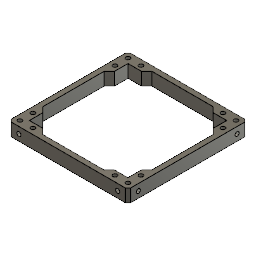
STRUCTURE UPPER FOSSASAT-1 v2 (Autodesk Fusion 360 design; units mm, degrees)
Autodesk Fusion 360 part; units mm, degrees
sketch "Sketch1" plane through (0, 0, 0) normal (0, 1, 0) x (1, 0, 0)
  line L0 (0, 0) -> (46, 0)
  line L1 (46, 0) -> (46, -46)
  line L2 (46, -46) -> (0, -46)
  line L3 (0, -46) -> (0, 0)
  line L4 (0, 0) -> (2, 0)
  line L5 (2, 0) -> (2, -2)
  circle A0 centre (2, -2) radius 0.8
  line L6 (5, -1.5) -> (5, -1)
  line L7 (23, 0) -> (23, -46)
  line L8 (23, -23) -> (42, -23)
  line L9 (42, -23) -> (42, -4)
  line L10 (42, -4) -> (4, -4)
  line L11 (4, -4) -> (4, -42)
  line L12 (4, -42) -> (42, -42)
  line L13 (42, -42) -> (42, -4)
  line L14 (0, -46) -> (2, -46)
  line L15 (2, -46) -> (2, -44)
  circle A1 centre (2, -44) radius 0.8
  line L16 (46, -46) -> (44, -46)
  line L17 (44, -46) -> (44, -44)
  circle A2 centre (44, -44) radius 0.8
  line L18 (46, 0) -> (44, 0)
  line L19 (44, 0) -> (44, -2)
  circle A3 centre (44, -2) radius 0.8
  line L20 (42, -4) -> (45.9628, -7.9628)
  line L21 (42, -4) -> (47.6042, -4) construction
  line L22 (42, -4) -> (38, 0)
  line L23 (42, -42) -> (46, -38)
  line L24 (46, -38) -> (38, -46)
  line L25 (4, -42) -> (8, -46)
  line L26 (8, -46) -> (0, -38)
  line L27 (4, -4) -> (8, 0)
  line L28 (8, 0) -> (0, -8)
  line L29 (2, -39) -> (2, -41)
  line L30 (2, -41) -> (2, -4)
  line L31 (5.0409, -2) -> (42, -2)
  line L32 (4, -44) -> (42, -44)
  line L33 (44, -40.936) -> (44, -4)
  dimension "d1" = 46
  dimension "d2" = 2
  dimension "d3" = 19
  dimension "d4" = 19
  dimension "d5" = 38
  dimension "d6" = 38
  dimension "d7" = 1.6
  dimension "d8" = 2
  dimension "d9" = 45
  measures "d4" distance of L0.start
  measures "d6" distance of L0.start
  measures "d7" diameter of A2
  measures "d9" angle of L20 L21
extrude "Extrude1" add sketch "Sketch1" along normal blind 6 contours L0 L3 L4 L27 L28 | L3 L26 L28 L29 L30 | L0 L7 L27 L28 L31 | L2 L3 L14 L25 L26 | L0 L7 L22 L31 | L0 L1 L18 L20 L22 L23 L24 L33 | L2 L7 L25 L26 L32 | L2 L7 L24 L32 | L1 L2 L16 L23 L24
extrude "Extrude2" cut 1 faces at (45.3333, 6, 14.6667) along direction (0, -1, 0) blind 1
chamfer "Chamfer1" distance 1 angle 45 4 edges at (46, 2.5, 46) (0, 2.5, 46) (46, 2.5, 0) (0, 2.5, 0)
sketch "Sketch2" plane through (0, 0, 0) normal (0, 0, -1) x (-1, 0, 0)
  line L0 (-1, 0) -> (-1, 5)
  line L1 (-1, 5) -> (-45, 5)
  line L2 (-45, 5) -> (-45, 0)
  line L3 (-45, 0) -> (-1, 0)
  line L4 (0, 0) -> (0, 5)
  line L5 (0, 2.5) -> (-4, 2.5)
  circle A0 centre (-4, 2.5) radius 0.8
  line L6 (-46, 5) -> (-46, 0)
  line L7 (-46, 2.5) -> (-42, 2.5)
  circle A1 centre (-42, 2.5) radius 0.8
  dimension "d15" = 1.6
  dimension "d16" = 4
  dimension "d17" = 1.6
  measures "d15" diameter of A0
  measures "d17" diameter of A1
extrude "Extrude3" cut sketch "Sketch2" against normal blind 3 contours A0 | A1
sketch "Sketch3" plane through (0, 0, 0) normal (-1, 0, 0) x (0, 0, 1)
  line L0 (1, 5) -> (1, 0)
  line L1 (1, 0) -> (45, 0)
  line L2 (45, 0) -> (45, 5)
  line L3 (45, 5) -> (1, 5)
  line L4 (0, 2.5) -> (4, 2.5)
  line L5 (46, 5) -> (46, 0)
  line L6 (46, 2.5) -> (42, 2.5)
  circle A0 centre (42, 2.5) radius 0.8
  circle A1 centre (4, 2.5) radius 0.8
  dimension "d20" = 4
  dimension "d21" = 1.6
  dimension "d22" = 1.6
  measures "d21" diameter of A0
  measures "d22" diameter of A1
extrude "Extrude4" cut sketch "Sketch3" against normal blind 3 contours A0 | A1
sketch "Sketch4" plane through (0, 0, 46) normal (0, 0, 1) x (1, 0, 0)
  line L0 (1, 5) -> (1, 0)
  line L1 (1, 0) -> (45, 0)
  line L2 (45, 0) -> (45, 5)
  line L3 (45, 5) -> (1, 5)
  line L4 (0, 2.5) -> (4, 2.5)
  circle A0 centre (4, 2.5) radius 0.8
  line L5 (46, 0) -> (46, 5)
  line L6 (42, 0) -> (42, 5)
  line L7 (46, 2.5) -> (42, 2.5)
  circle A1 centre (42, 2.5) radius 0.8
  dimension "d25" = 1.6
  dimension "d26" = 1.6
  measures "d25" diameter of A0
  measures "d26" diameter of A1
extrude "Extrude5" cut sketch "Sketch4" against normal blind 1.6 contours L6 L7 A1 | L6 A1 | L6 L7 A1 | A0
sketch "Sketch5" plane through (46, 0, 0) normal (1, 0, 0) x (0, 0, -1)
  line L0 (-1, 0) -> (-1, 5)
  line L1 (-1, 5) -> (-45, 5)
  line L2 (-45, 5) -> (-45, 0)
  line L3 (-45, 0) -> (-1, 0)
  line L4 (-46, 2.5) -> (-42, 2.5)
  circle A0 centre (-42, 2.5) radius 0.8
  line L5 (0, 2.5) -> (-4, 2.5)
  circle A1 centre (-4, 2.5) radius 0.8
  dimension "d29" = 4
  dimension "d30" = 1.6
  measures "d30" diameter of A1
extrude "Extrude6" cut sketch "Sketch5" against normal blind 3 contours A0 | A1
extrude "Extrude7" cut 2 faces at (4.3142, 2.6814, 44.4) (42.1333, 2.9623, 44.4) along direction (0, 0, -1) blind 1.4
sketch "Sketch6" plane through (0, 5, 0) normal (0, 1, 0) x (-1, 0, 0)
  circle A0 centre (-2, 2) radius 0.8
  circle A1 centre (-2, 44) radius 0.8
  circle A2 centre (-44, 2) radius 0.8
  circle A3 centre (-44, 44) radius 0.8
  line L0 (-40, 2) -> (-42, 4)
  line L1 (-42, 4) -> (-44, 6)
  line L2 (-44, 6) -> (-44, 40)
  line L3 (-44, 40) -> (-40, 44)
  line L4 (-40, 44) -> (-6, 44)
  line L5 (-6, 44) -> (-2, 40)
  line L6 (-2, 40) -> (-2, 6)
  line L7 (-2, 6) -> (-6, 2)
  line L8 (-6, 2) -> (-40, 2)
  line L9 (-1, 0) -> (0, 1)
  line L10 (0, 1) -> (0, 45)
  line L11 (0, 45) -> (-1, 46)
  line L12 (-1, 46) -> (-45, 46)
  line L13 (-45, 46) -> (-46, 45)
  line L14 (-46, 45) -> (-46, 1)
  line L15 (-46, 1) -> (-45, 0)
  line L16 (-45, 0) -> (-1, 0)
  line L17 (-46, 38.6089) -> (-43.8, 38.6089)
  line L18 (-44, 44) -> (-42, 44)
  line L19 (-43.8, 38.6089) -> (-43.8, 44)
  line L20 (-43.8, 44) -> (-43.8, 39)
  line L21 (-23, 23) -> (-23, 42)
  line L22 (-23, 42) -> (-42, 42)
  line L23 (-42, 42) -> (-42, 4)
  line L24 (-42, 4) -> (-4, 4)
  line L25 (-4, 4) -> (-4, 42)
  line L26 (-4, 42) -> (-23, 42)
  circle A4 centre (-43.8, 38.6089) radius 0.8
  line L27 (-43.8, 38.6089) -> (-43.8, 36.6089)
  line L28 (-43.8, 36.6089) -> (-42, 36.6089)
  line L29 (-42, 36.6089) -> (-46.5, 36.6089)
  line L30 (-42, 36.6089) -> (-44, 34.6089)
  line L31 (-42, 36.6089) -> (-39.1716, 36.6089) construction
  circle A5 centre (-44, 44) radius 0.8
  dimension "d35" = 1.6
  dimension "d36" = 135
  measures "d35" diameter of A4
  measures "d36" angle of L30 L31
extrude "Extrude8" add sketch "Sketch6" against normal blind 5 contours A0 | A1 | A2 | A3 L18 L19 L20 A5 | A3 L18 L19 L20 A5
sketch "Sketch7" plane through (0, 5, 0) normal (0, 1, 0) x (-1, 0, 0)
  line L0 (-40, 2) -> (-42, 4)
  line L1 (-42, 4) -> (-44, 6)
  line L2 (-44, 6) -> (-44, 40)
  line L3 (-44, 40) -> (-40, 44)
  line L4 (-40, 44) -> (-6, 44)
  line L5 (-6, 44) -> (-2, 40)
  line L6 (-2, 40) -> (-2, 6)
  line L7 (-2, 6) -> (-6, 2)
  line L8 (-6, 2) -> (-40, 2)
  line L9 (-1, 0) -> (0, 1)
  line L10 (0, 1) -> (0, 45)
  line L11 (0, 45) -> (-1, 46)
  line L12 (-1, 46) -> (-45, 46)
  line L13 (-45, 46) -> (-46, 45)
  line L14 (-46, 45) -> (-46, 1)
  line L15 (-46, 1) -> (-45, 0)
  line L16 (-45, 0) -> (-1, 0)
  line L17 (0, 0) -> (-2.2, 0)
  line L18 (-2.2, 0) -> (-2.2, 2.2)
  circle A0 centre (-2.2, 2.2) radius 0.8
  line L19 (-2.2, 2.2) -> (-2.2, 7.2)
  circle A1 centre (-2.2, 7.2) radius 0.8
  line L20 (-2.2, 2.2) -> (-7.2, 2.2)
  circle A2 centre (-7.2, 2.2) radius 0.8
  line L21 (-2.2, 7.2) -> (-2.2, 9.2)
  line L22 (-7.2, 2.2) -> (-9.2, 2.2)
  line L23 (-23, 23) -> (-23, 4)
  line L24 (-23, 4) -> (-4, 4)
  line L25 (-4, 4) -> (-4, 42)
  line L26 (-4, 42) -> (-42, 42)
  line L27 (-42, 42) -> (-42, 4)
  line L28 (-42, 4) -> (-23, 4)
  line L29 (-2.2, 9.2) -> (-4, 9.2)
  line L30 (-2.2, 9.2) -> (-1.6806, 9.2)
  line L31 (-9.2, 2.2) -> (-9.2, 4)
  line L32 (-9.2, 2.2) -> (-9.2, 1.7812)
  line L33 (-4, 9.2) -> (-2, 11.2)
  line L34 (-4, 9.2) -> (-1.1716, 9.2) construction
  line L35 (-9.2, 4) -> (-11.2, 2)
  line L36 (-46, 0) -> (-43.8, 0)
  line L37 (-43.8, 0) -> (-43.8, 2.2)
  circle A3 centre (-43.8, 2.2) radius 0.8
  line L38 (-43.8, 2.2) -> (-38.8, 2.2)
  line L39 (-43.8, 2.2) -> (-43.8, 7.2)
  circle A4 centre (-38.8, 2.2) radius 0.8
  circle A5 centre (-43.8, 7.2) radius 0.8
  line L40 (-43.8, 7.2) -> (-43.8, 9.2)
  line L41 (-38.8, 2.2) -> (-36.8, 2.2)
  line L42 (-43.8, 9.2) -> (-44.3378, 9.2)
  line L43 (-44.3378, 9.2) -> (-42, 9.2)
  line L44 (-36.8, 2.2) -> (-36.8, 1.5)
  line L45 (-36.8, 1.5) -> (-36.8, 4)
  line L46 (-36.8, 4) -> (-34.8, 2)
  line L47 (-36.8, 4) -> (-33.9716, 4) construction
  line L48 (-42, 9.2) -> (-44, 11.2)
  line L49 (-42, 9.2) -> (-39.1716, 9.2) construction
  line L50 (0, 46) -> (-2.2, 46)
  line L51 (-2.2, 46) -> (-2.2, 43.8)
  circle A6 centre (-2.2, 43.8) radius 0.8
  line L52 (-2.2, 43.8) -> (-7.2, 43.8)
  line L53 (-2.2, 43.8) -> (-2.2, 38.8)
  circle A7 centre (-7.2, 43.8) radius 0.8
  circle A8 centre (-2.2, 38.8) radius 0.8
  line L54 (-7.2, 43.8) -> (-9.2, 43.8)
  line L55 (-2.2, 38.8) -> (-2.2, 36.8)
  line L56 (-9.2, 43.8) -> (-9.2, 44.5)
  line L57 (-2.2, 36.8) -> (-1.5, 36.8)
  line L58 (-2, 36.8) -> (-4, 36.8)
  line L59 (-9.2, 44) -> (-9.2, 42)
  line L60 (-9.2, 42) -> (-11.2, 44)
  line L61 (-4, 36.8) -> (-2, 34.8)
  line L62 (-46, 46) -> (-43.8, 46)
  line L63 (-43.8, 46) -> (-43.8, 43.8)
  circle A9 centre (-43.8, 43.8) radius 0.8
  line L64 (-43.8, 43.8) -> (-43.8, 38.8)
  line L65 (-43.8, 43.8) -> (-38.8, 43.8)
  circle A10 centre (-43.8, 38.8) radius 0.8
  circle A11 centre (-38.8, 43.8) radius 0.8
  line L66 (-43.8, 38.8) -> (-43.8, 36.8)
  line L67 (-38.8, 43.8) -> (-36.8, 43.8)
  line L68 (-36.8, 43.8) -> (-36.8, 45)
  line L69 (-43.8, 36.8) -> (-45, 36.8)
  line L70 (-43.8, 36.8) -> (-42, 36.8)
  line L71 (-36.8, 43.8) -> (-36.8, 42)
  line L72 (-42, 36.8) -> (-44, 34.8)
  line L73 (-42, 36.8) -> (-39.1716, 36.8) construction
  line L74 (-36.8, 42) -> (-34.8, 44)
  dimension "d39" = 1.6
  dimension "d40" = 1.6
  dimension "d41" = 5
  dimension "d42" = 1.6
  dimension "d43" = 2
  dimension "d44" = 2
  dimension "d45" = 45
  dimension "d46" = 135
  dimension "d47" = 1.6
  dimension "d48" = 1.6
  dimension "d49" = 1.6
  dimension "d50" = 45
  dimension "d51" = 135
  dimension "d53" = 2.2
  dimension "d54" = 1.6
  dimension "d55" = 5
  dimension "d56" = 1.6
  dimension "d57" = 1.6
  dimension "d58" = 2
  dimension "d59" = 2.2
  dimension "d60" = 1.6
  dimension "d61" = 5
  dimension "d62" = 1.6
  dimension "d63" = 1.6
  dimension "d64" = 135
  dimension "d65" = 45
  measures "d39" diameter of A0
  measures "d40" diameter of A1
  measures "d42" diameter of A2
  measures "d45" angle of L33 L34
  measures "d46" angle of L34 L35
  measures "d47" diameter of A3
  measures "d48" diameter of A4
  measures "d49" diameter of A5
  measures "d50" angle of L46 L47
  measures "d51" angle of L48 L49
  measures "d54" diameter of A6
  measures "d56" diameter of A7
  measures "d57" diameter of A8
  measures "d60" diameter of A9
  measures "d62" diameter of A10
  measures "d63" diameter of A11
  measures "d64" angle of L72 L73
  measures "d65" angle of L73 L74
extrude "Extrude9" add sketch "Sketch7" against normal blind 5 contours L0 L8 L38 A4 | L0 L28 L38 A4 L41 L45 | L1 L27 L39 A5 L40 L43 | L8 A4 L41 L44 L45 | L1 L2 L39 A5 | L2 L42 L43 L48 | L8 L44 L45 L46 | L3 L27 L64 A10 L66 L70 | L2 L69 L70 L72 | L2 A5 L40 L42 L43 | L3 L26 L65 A11 L67 L71 | L2 A10 L66 L69 | L7 L20 A2 L22 L24 L31 | L8 L31 L32 L35 | L2 L3 L64 A10 | L3 L4 L65 A11 | L4 L68 L71 L74 | L7 L19 A1 L21 L25 L29 | L8 A2 L22 L32 | L5 L26 L52 A7 L54 L59 | L4 L56 L59 L60 | L4 A11 L67 L68 | L6 L7 L19 A1 | L7 L8 L20 A2 | L6 L29 L30 L33 | L5 L25 L53 A8 L55 L58 | L4 A7 L54 L56 L59 | L6 L57 L58 L61 | L6 A1 L21 L30 | L4 L5 L52 A7 | L5 L6 L53 A8 | L6 A8 L55 L57 L58
sketch "Sketch8" plane through (0, 5, 0) normal (0, 1, 0) x (-1, 0, 0)
  line L0 (-38.0254, 2) -> (-39.5746, 2)
  arc A0 (-38.0254, 2) -> (-39.5746, 2) centre (-38.8, 2.2) ccw
  line L1 (-34.8, 2) -> (-36.8, 4)
  line L2 (-36.8, 4) -> (-42, 4)
  line L3 (-42, 4) -> (-42, 9.2)
  line L4 (-42, 9.2) -> (-44, 11.2)
  line L5 (-44, 11.2) -> (-44, 34.8)
  line L6 (-44, 34.8) -> (-42, 36.8)
  line L7 (-42, 36.8) -> (-42, 42)
  line L8 (-42, 42) -> (-36.8, 42)
  line L9 (-36.8, 42) -> (-34.8, 44)
  line L10 (-34.8, 44) -> (-11.2, 44)
  line L11 (-11.2, 44) -> (-9.2, 42)
  line L12 (-9.2, 42) -> (-4, 42)
  line L13 (-4, 42) -> (-4, 36.8)
  line L14 (-4, 36.8) -> (-2, 34.8)
  line L15 (-2, 34.8) -> (-2, 11.2)
  line L16 (-2, 11.2) -> (-4, 9.2)
  line L17 (-4, 9.2) -> (-4, 4)
  line L18 (-4, 4) -> (-9.2, 4)
  line L19 (-9.2, 4) -> (-11.2, 2)
  line L20 (-11.2, 2) -> (-34.8, 2)
  arc A1 (-44, 6.4254) -> (-44, 7.9746) centre (-43.8, 7.2) ccw
  line L21 (-44, 6.4254) -> (-44, 7.9746)
  arc A2 (-6.4254, 2) -> (-7.9746, 2) centre (-7.2, 2.2) ccw
  line L22 (-6.4254, 2) -> (-7.9746, 2)
  line L23 (-7.9746, 44) -> (-6.4254, 44)
  arc A3 (-7.9746, 44) -> (-6.4254, 44) centre (-7.2, 43.8) ccw
  arc A4 (-2, 7.9746) -> (-2, 6.4254) centre (-2.2, 7.2) ccw
  line L24 (-2, 7.9746) -> (-2, 6.4254)
  line L25 (-44, 38.0254) -> (-44, 39.5746)
  arc A5 (-44, 38.0254) -> (-44, 39.5746) centre (-43.8, 38.8) ccw
  arc A6 (-2, 39.5746) -> (-2, 38.0254) centre (-2.2, 38.8) ccw
  line L26 (-2, 39.5746) -> (-2, 38.0254)
  arc A7 (-39.5746, 44) -> (-38.0254, 44) centre (-38.8, 43.8) ccw
  line L27 (-39.5746, 44) -> (-38.0254, 44)
  line L28 (-1, 0) -> (0, 1)
  line L29 (0, 1) -> (0, 45)
  line L30 (0, 45) -> (-1, 46)
  line L31 (-1, 46) -> (-45, 46)
  line L32 (-45, 46) -> (-46, 45)
  line L33 (-46, 45) -> (-46, 1)
  line L34 (-46, 1) -> (-45, 0)
  line L35 (-45, 0) -> (-1, 0)
  circle A8 centre (-38.8, 2.2) radius 0.8
  circle A9 centre (-43.8, 7.2) radius 0.8
  circle A10 centre (-38.8, 43.8) radius 0.8
  circle A11 centre (-43.8, 38.8) radius 0.8
  circle A12 centre (-7.2, 43.8) radius 0.8
  circle A13 centre (-2.2, 38.8) radius 0.8
  circle A14 centre (-7.2, 2.2) radius 0.8
  circle A15 centre (-2.2, 7.2) radius 0.8
  line L36 (-2.2, 7.2) -> (-2.2, 2.2)
  circle A16 centre (-2.2, 2.2) radius 0.8
  line L37 (-43.8, 38.8) -> (-43.8, 43.8)
  circle A17 centre (-43.8, 43.8) radius 0.8
  line L38 (-2.2, 38.8) -> (-2.2, 43.8)
  line L39 (-2.2, 43.8) -> (-7.2, 43.8)
  circle A18 centre (-2.2, 43.8) radius 0.8
  line L40 (-38.8, 2.2) -> (-43.8, 2.2)
  circle A19 centre (-43.8, 2.2) radius 0.8
extrude "Extrude10" cut sketch "Sketch8" against normal blind 5 contours L0 A8 | L21 A9 | L22 A14 | L23 A12 | L24 A15 | L25 A11 | L26 A13 | L27 A10 | A16 | A17 | L38 L39 A18 | L38 L39 A18 | A19
